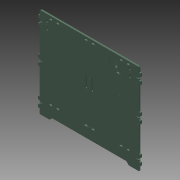
# Autodesk Inventor part: tyl_gt2
Saved by Autodesk Inventor 2013 (Build 170138000, 138)
## iProperties
Created: 2014-01-09
Part Number: tyl_gt2
Material: Generic
Document SubType Name: Modeling
Designer: dzban
Density: 1 g/cm^3
Author: dzban
Autodesk Inventor part; units mm, degrees
ref_plane "YZ Plane" through (0, 0, 0) normal (1, 0, 0) x (0, 1, 0)
ref_plane "XZ Plane" through (0, 0, 0) normal (0, 1, 0) x (-1, 0, 0)
ref_plane "XY Plane" through (0, 0, 0) normal (0, 0, 1) x (1, 0, 0)
sketch "Sketch1" plane through (0, 0, 0) normal (0, 1, 0) x (-1, 0, 0)
  line L0 (126.9556, -58.4026) -> (126.9556, -52.0026)
  line L1 (126.9556, -52.0026) -> (138.8556, -52.0026)
  line L2 (138.8556, -52.0026) -> (138.8556, -58.4026)
  line L3 (138.8556, -58.4026) -> (126.9556, -58.4026)
  arc A0 (161.4486, -20.0075) -> (158.9486, -20.0075) centre (160.1986, -20.0075) ccw
  line L4 (161.4486, -20.0075) -> (161.4486, -40.0075)
  arc A1 (158.9486, -40.0075) -> (161.4486, -40.0075) centre (160.1986, -40.0075) ccw
  line L5 (158.9486, -40.0075) -> (158.9486, -20.0075)
  arc A2 (168.4486, -40.0075) -> (170.9486, -40.0075) centre (169.6986, -40.0075) ccw
  line L6 (168.4486, -40.0075) -> (168.4486, -20.0075)
  arc A3 (170.9486, -20.0075) -> (168.4486, -20.0075) centre (169.6986, -20.0075) ccw
  line L7 (170.9486, -20.0075) -> (170.9486, -40.0075)
  line L8 (261.2986, -171.5221) -> (254.8986, -171.5221)
  line L9 (254.8986, -171.5221) -> (254.8986, -125.0075)
  line L10 (254.8986, -125.0075) -> (261.2986, -125.0075)
  line L11 (261.2986, -125.0075) -> (261.2986, -171.5221)
  line L12 (230.8986, -171.5221) -> (230.8986, -125.0075)
  line L13 (230.8986, -125.0075) -> (237.2986, -125.0075)
  line L14 (237.2986, -125.0075) -> (237.2986, -171.5221)
  line L15 (237.2986, -171.5221) -> (230.8986, -171.5221)
  line L16 (378.2986, -8.4075) -> (366.2986, -8.4075)
  line L17 (366.2986, -8.4075) -> (366.2986, -2.0075)
  line L18 (366.2986, -2.0075) -> (378.2986, -2.0075)
  line L19 (378.2986, -2.0075) -> (378.2986, -8.4075)
  line L20 (405.8986, -8.4075) -> (393.8986, -8.4075)
  line L21 (393.8986, -8.4075) -> (393.8986, -2.0075)
  line L22 (393.8986, -2.0075) -> (405.8986, -2.0075)
  line L23 (405.8986, -2.0075) -> (405.8986, -8.4075)
  line L24 (238.2986, -8.4075) -> (226.2986, -8.4075)
  line L25 (226.2986, -8.4075) -> (226.2986, -2.0075)
  line L26 (226.2986, -2.0075) -> (238.2986, -2.0075)
  line L27 (238.2986, -2.0075) -> (238.2986, -8.4075)
  line L28 (265.8986, -8.4075) -> (253.8986, -8.4075)
  line L29 (253.8986, -8.4075) -> (253.8986, -2.0075)
  line L30 (253.8986, -2.0075) -> (265.8986, -2.0075)
  line L31 (265.8986, -2.0075) -> (265.8986, -8.4075)
  line L32 (98.2986, -8.4075) -> (86.2986, -8.4075)
  line L33 (86.2986, -8.4075) -> (86.2986, -2.0075)
  line L34 (86.2986, -2.0075) -> (98.2986, -2.0075)
  line L35 (98.2986, -2.0075) -> (98.2986, -8.4075)
  line L36 (125.8986, -8.4075) -> (113.8986, -8.4075)
  line L37 (113.8986, -8.4075) -> (113.8986, -2.0075)
  line L38 (113.8986, -2.0075) -> (125.8986, -2.0075)
  line L39 (125.8986, -2.0075) -> (125.8986, -8.4075)
  line L40 (378.2986, -303.4075) -> (366.2986, -303.4075)
  line L41 (366.2986, -303.4075) -> (366.2986, -297.0075)
  line L42 (366.2986, -297.0075) -> (378.2986, -297.0075)
  line L43 (378.2986, -297.0075) -> (378.2986, -303.4075)
  line L44 (405.8986, -303.4075) -> (393.8986, -303.4075)
  line L45 (393.8986, -303.4075) -> (393.8986, -297.0075)
  line L46 (393.8986, -297.0075) -> (405.8986, -297.0075)
  line L47 (405.8986, -297.0075) -> (405.8986, -303.4075)
  line L48 (238.2986, -303.4075) -> (226.2986, -303.4075)
  line L49 (226.2986, -303.4075) -> (226.2986, -297.0075)
  line L50 (226.2986, -297.0075) -> (238.2986, -297.0075)
  line L51 (238.2986, -297.0075) -> (238.2986, -303.4075)
  line L52 (265.8986, -303.4075) -> (253.8986, -303.4075)
  line L53 (253.8986, -303.4075) -> (253.8986, -297.0075)
  line L54 (253.8986, -297.0075) -> (265.8986, -297.0075)
  line L55 (265.8986, -297.0075) -> (265.8986, -303.4075)
  line L56 (98.2986, -303.4075) -> (86.2986, -303.4075)
  line L57 (86.2986, -303.4075) -> (86.2986, -297.0075)
  line L58 (86.2986, -297.0075) -> (98.2986, -297.0075)
  line L59 (98.2986, -297.0075) -> (98.2986, -303.4075)
  line L60 (125.8986, -303.4075) -> (113.8986, -303.4075)
  line L61 (113.8986, -303.4075) -> (113.8986, -297.0075)
  line L62 (113.8986, -297.0075) -> (125.8986, -297.0075)
  line L63 (125.8986, -297.0075) -> (125.8986, -303.4075)
  line L64 (443.6986, -314.9075) -> (436.6986, -314.9075)
  line L65 (436.6986, -314.9075) -> (436.6986, -316.1575)
  line L66 (436.6986, -316.1575) -> (434.8986, -316.1575)
  line L67 (434.8986, -316.1575) -> (434.8986, -314.9075)
  line L68 (434.8986, -314.9075) -> (433.0986, -314.9075)
  line L69 (433.0986, -314.9075) -> (433.0986, -311.9075)
  line L70 (433.0986, -311.9075) -> (434.8986, -311.9075)
  line L71 (434.8986, -311.9075) -> (434.8986, -310.6575)
  line L72 (434.8986, -310.6575) -> (436.6986, -310.6575)
  line L73 (436.6986, -310.6575) -> (436.6986, -311.9075)
  line L74 (436.6986, -311.9075) -> (443.6986, -311.9075)
  line L75 (443.6986, -311.9075) -> (443.6986, -305.8075)
  line L76 (443.6986, -305.8075) -> (449.6986, -305.5075)
  line L77 (449.6986, -305.5075) -> (449.6986, -293.7075)
  line L78 (449.6986, -293.7075) -> (443.6986, -293.4075)
  line L79 (443.6986, -293.4075) -> (443.6986, -189.0075)
  line L80 (443.6986, -189.0075) -> (449.6986, -188.7075)
  line L81 (449.6986, -188.7075) -> (449.6986, -176.9075)
  line L82 (449.6986, -176.9075) -> (443.6986, -176.6075)
  line L83 (443.6986, -176.6075) -> (443.6986, -170.5075)
  line L84 (443.6986, -170.5075) -> (436.6986, -170.5075)
  line L85 (436.6986, -170.5075) -> (436.6986, -171.7575)
  line L86 (436.6986, -171.7575) -> (434.8986, -171.7575)
  line L87 (434.8986, -171.7575) -> (434.8986, -170.5075)
  line L88 (434.8986, -170.5075) -> (433.0986, -170.5075)
  line L89 (433.0986, -170.5075) -> (433.0986, -167.5075)
  line L90 (433.0986, -167.5075) -> (434.8986, -167.5075)
  line L91 (434.8986, -167.5075) -> (434.8986, -166.2575)
  line L92 (434.8986, -166.2575) -> (436.6986, -166.2575)
  line L93 (436.6986, -166.2575) -> (436.6986, -167.5075)
  line L94 (436.6986, -167.5075) -> (443.6986, -167.5075)
  line L95 (443.6986, -167.5075) -> (443.6986, -161.4075)
  line L96 (443.6986, -161.4075) -> (449.6986, -161.1075)
  line L97 (449.6986, -161.1075) -> (449.6986, -149.3075)
  line L98 (449.6986, -149.3075) -> (443.6986, -149.0075)
  line L99 (443.6986, -149.0075) -> (443.6986, -54.0075)
  line L100 (443.6986, -54.0075) -> (449.6986, -53.7075)
  line L101 (449.6986, -53.7075) -> (449.6986, -41.9075)
  line L102 (449.6986, -41.9075) -> (443.6986, -41.6075)
  line L103 (443.6986, -41.6075) -> (443.6986, -35.5075)
  line L104 (443.6986, -35.5075) -> (436.6986, -35.5075)
  line L105 (436.6986, -35.5075) -> (436.6986, -36.7575)
  line L106 (436.6986, -36.7575) -> (434.8986, -36.7575)
  line L107 (434.8986, -36.7575) -> (434.8986, -35.5075)
  line L108 (434.8986, -35.5075) -> (433.0986, -35.5075)
  line L109 (433.0986, -35.5075) -> (433.0986, -32.5075)
  line L110 (433.0986, -32.5075) -> (434.8986, -32.5075)
  line L111 (434.8986, -32.5075) -> (434.8986, -31.2575)
  line L112 (434.8986, -31.2575) -> (436.6986, -31.2575)
  line L113 (436.6986, -31.2575) -> (436.6986, -32.5075)
  line L114 (436.6986, -32.5075) -> (443.6986, -32.5075)
  line L115 (443.6986, -32.5075) -> (443.6986, -26.4075)
  line L116 (443.6986, -26.4075) -> (449.6986, -26.1075)
  line L117 (449.6986, -26.1075) -> (449.6986, -14.3075)
  line L118 (449.6986, -14.3075) -> (443.6986, -14.0075)
  line L119 (443.6986, -14.0075) -> (443.6986, 0.9925)
  arc A4 (443.6986, 0.9925) -> (438.6986, 5.9925) centre (438.6986, 0.9925) ccw
  line L120 (438.6986, 5.9925) -> (53.4986, 5.9925)
  arc A5 (53.4986, 5.9925) -> (48.4986, 0.9925) centre (53.4986, 0.9925) ccw
  line L121 (48.4986, 0.9925) -> (48.4986, -14.0075)
  line L122 (48.4986, -14.0075) -> (42.4986, -14.3075)
  line L123 (42.4986, -14.3075) -> (42.4986, -26.1075)
  line L124 (42.4986, -26.1075) -> (48.4986, -26.4075)
  line L125 (48.4986, -26.4075) -> (48.4986, -32.5075)
  line L126 (48.4986, -32.5075) -> (55.4986, -32.5075)
  line L127 (55.4986, -32.5075) -> (55.4986, -31.2575)
  line L128 (55.4986, -31.2575) -> (57.2986, -31.2575)
  line L129 (57.2986, -31.2575) -> (57.2986, -32.5075)
  line L130 (57.2986, -32.5075) -> (59.0986, -32.5075)
  line L131 (59.0986, -32.5075) -> (59.0986, -35.5075)
  line L132 (59.0986, -35.5075) -> (57.2986, -35.5075)
  line L133 (57.2986, -35.5075) -> (57.2986, -36.7575)
  line L134 (57.2986, -36.7575) -> (55.4986, -36.7575)
  line L135 (55.4986, -36.7575) -> (55.4986, -35.5075)
  line L136 (55.4986, -35.5075) -> (48.4986, -35.5075)
  line L137 (48.4986, -35.5075) -> (48.4986, -41.6075)
  line L138 (48.4986, -41.6075) -> (42.4986, -41.9075)
  line L139 (42.4986, -41.9075) -> (42.4986, -53.7075)
  line L140 (42.4986, -53.7075) -> (48.4986, -54.0075)
  line L141 (48.4986, -54.0075) -> (48.4986, -149.0075)
  line L142 (48.4986, -149.0075) -> (42.4986, -149.3075)
  line L143 (42.4986, -149.3075) -> (42.4986, -161.1075)
  line L144 (42.4986, -161.1075) -> (48.4986, -161.4075)
  line L145 (48.4986, -161.4075) -> (48.4986, -167.5075)
  line L146 (48.4986, -167.5075) -> (55.4986, -167.5075)
  line L147 (55.4986, -167.5075) -> (55.4986, -166.2575)
  line L148 (55.4986, -166.2575) -> (57.2986, -166.2575)
  line L149 (57.2986, -166.2575) -> (57.2986, -167.5075)
  line L150 (57.2986, -167.5075) -> (59.0986, -167.5075)
  line L151 (59.0986, -167.5075) -> (59.0986, -170.5075)
  line L152 (59.0986, -170.5075) -> (57.2986, -170.5075)
  line L153 (57.2986, -170.5075) -> (57.2986, -171.7575)
  line L154 (57.2986, -171.7575) -> (55.4986, -171.7575)
  line L155 (55.4986, -171.7575) -> (55.4986, -170.5075)
  line L156 (55.4986, -170.5075) -> (48.4986, -170.5075)
  line L157 (48.4986, -170.5075) -> (48.4986, -176.6075)
  line L158 (48.4986, -176.6075) -> (42.4986, -176.9075)
  line L159 (42.4986, -176.9075) -> (42.4986, -188.7075)
  line L160 (42.4986, -188.7075) -> (48.4986, -189.0075)
  line L161 (48.4986, -189.0075) -> (48.4986, -293.4075)
  line L162 (48.4986, -293.4075) -> (42.4986, -293.7075)
  line L163 (42.4986, -293.7075) -> (42.4986, -305.5075)
  line L164 (42.4986, -305.5075) -> (48.4986, -305.8075)
  line L165 (48.4986, -305.8075) -> (48.4986, -311.9075)
  line L166 (48.4986, -311.9075) -> (55.4986, -311.9075)
  line L167 (55.4986, -311.9075) -> (55.4986, -310.6575)
  line L168 (55.4986, -310.6575) -> (57.2986, -310.6575)
  line L169 (57.2986, -310.6575) -> (57.2986, -311.9075)
  line L170 (57.2986, -311.9075) -> (59.0986, -311.9075)
  line L171 (59.0986, -311.9075) -> (59.0986, -314.9075)
  line L172 (59.0986, -314.9075) -> (57.2986, -314.9075)
  line L173 (57.2986, -314.9075) -> (57.2986, -316.1575)
  line L174 (57.2986, -316.1575) -> (55.4986, -316.1575)
  line L175 (55.4986, -316.1575) -> (55.4986, -314.9075)
  line L176 (55.4986, -314.9075) -> (48.4986, -314.9075)
  line L177 (48.4986, -314.9075) -> (48.4986, -321.0075)
  line L178 (48.4986, -321.0075) -> (42.4986, -321.3075)
  line L179 (42.4986, -321.3075) -> (42.4986, -333.1075)
  line L180 (42.4986, -333.1075) -> (48.4986, -333.4075)
  line L181 (48.4986, -333.4075) -> (48.4986, -353.4075)
  line L182 (48.4986, -353.4075) -> (88.4986, -353.4075)
  line L183 (88.4986, -353.4075) -> (98.4986, -343.4075)
  line L184 (98.4986, -343.4075) -> (393.6986, -343.4075)
  line L185 (393.6986, -343.4075) -> (403.6986, -353.4075)
  line L186 (403.6986, -353.4075) -> (443.6986, -353.4075)
  line L187 (443.6986, -353.4075) -> (443.6986, -333.4075)
  line L188 (443.6986, -333.4075) -> (449.6986, -333.1075)
  line L189 (449.6986, -333.1075) -> (449.6986, -321.3075)
  line L190 (449.6986, -321.3075) -> (443.6986, -321.0075)
  line L191 (443.6986, -321.0075) -> (443.6986, -314.9075)
  circle A6 centre (425.6986, -61.0075) radius 1.5
  circle A7 centre (66.4986, -61.0075) radius 1.5
  circle A8 centre (57.4986, -52.0075) radius 1.5
  circle A9 centre (434.6986, -52.0075) radius 1.5
  circle A10 centre (106.0986, -300.2075) radius 1.5
  circle A11 centre (246.0986, -300.2075) radius 1.5
  circle A12 centre (386.0986, -300.2075) radius 1.5
  circle A13 centre (106.0986, -5.2075) radius 1.5
  circle A14 centre (246.0986, -5.2075) radius 1.5
  circle A15 centre (386.0986, -5.2075) radius 1.5
  circle A16 centre (246.0986, -132.7575) radius 1.5
  circle A17 centre (246.0986, -154.2575) radius 1.5
  circle A18 centre (140.1628, -36.0853) radius 6
  circle A19 centre (122.9556, -55.2026) radius 1.5
  circle A20 centre (118.4986, -127.4183) radius 1.5
  circle A21 centre (136.1628, -24.0853) radius 1.5
  circle A22 centre (136.1628, -48.0853) radius 1.5
  circle A23 centre (55.4986, -192.4702) radius 1.5
  circle A24 centre (63.4986, -192.4702) radius 1.5
  circle A25 centre (144.1628, -48.0853) radius 1.5
  circle A26 centre (144.1628, -24.0853) radius 1.5
  circle A27 centre (124.9087, -130.187) radius 1.5
  point P0 (0, 0)
  dimension "d0" = 5.9925
  dimension "d1" = 48.4986
  dimension "d2" = 359.4
  dimension "d3" = 395.2
  dimension "d4" = 5
  dimension "d7" = 38.5
  dimension "d8" = 12.4
  dimension "d9" = 6.1
  dimension "d10" = 11.8
  dimension "d11" = 0.3
  dimension "d12" = 6
  dimension "d13" = 3
  dimension "d14" = 7
  dimension "d15" = 1.8
  dimension "d16" = 1.8
  dimension "d17" = 1.25
  dimension "d18" = 1.25
  dimension "d19" = 6.1
  dimension "d20" = 12.4
  dimension "d21" = 135
  dimension "d22" = 6.1
  dimension "d23" = 12.4
  dimension "d24" = 3
  dimension "d25" = 6.1
  dimension "d26" = 12.4
  dimension "d31" = 144.4
  dimension "d32" = 6.1
  dimension "d33" = 12.4
  dimension "d34" = 3
  dimension "d35" = 6.1
  dimension "d36" = 12.4
  dimension "d39" = 11.2
  dimension "d41" = 140
  dimension "d42" = 140
  dimension "d43" = 6.4
  dimension "d44" = 3.2
  dimension "d45" = 3
  dimension "d46" = 12
  dimension "d47" = 7.8
  dimension "d48" = 7.8
  dimension "d49" = 12
  dimension "d50" = 7.8
  dimension "d51" = 7.8
  dimension "d52" = 12
  dimension "d53" = 12
  dimension "d54" = 7.8
  dimension "d55" = 12
  dimension "d56" = 7.8
  dimension "d57" = 12
  dimension "d58" = 53.2
  dimension "d59" = 3.2
  dimension "d61" = 6.4
  dimension "d62" = 6.4
  dimension "d63" = 11.9
  dimension "d64" = 4
  dimension "d65" = 61.1951
  dimension "d66" = 74.457
  dimension "d67" = 3.2
  dimension "d68" = 8
  dimension "d69" = 24
  dimension "d70" = 30.0778
  dimension "d71" = 87.6641
  dimension "d72" = 4
  dimension "d73" = 12
  constraints: 384 end point, 125 parallel, 72 collinear, 28 centre point, 28 tangent, 24 equal radius, 12 point on circle, 11 horizontal alignment, 8 vertical alignment, 6 vertical, 4 horizontal, 1 perpendicular
  measures "d0" distance from line of point (0, 0) L120
  measures "d1" distance from line of point (0, 0) L121
  measures "d2" distance between parallel lines of L120 L182
  measures "d3" distance between parallel lines of L119 L121
  measures "d4" radius of A5
  measures "d7" distance between parallel lines of L120 L126
  measures "d8" distance of L121.end L124.end
  measures "d9" distance of L124.end L125.end
  measures "d10" distance of L122.end L123.end
  measures "d11" vertical distance of L121.end L122.end
  measures "d12" distance between parallel lines of L121 L123
  measures "d13" distance between parallel lines of L126 L136
  measures "d14" distance between parallel lines of L135 L137
  measures "d15" distance from line of L132.end L135
  measures "d16" distance between parallel lines of L131 L133
  measures "d17" distance between parallel lines of L128 L130
  measures "d18" distance between parallel lines of L132 L134
  measures "d19" distance of L136.end L137.end
  measures "d20" distance of L137.end L140.end
  measures "d21" distance between parallel lines of L146 L126
  measures "d22" distance of L144.end L145.end
  measures "d23" distance of L141.end L144.end
  measures "d24" distance between parallel lines of L146 L156
  measures "d25" distance of L156.end L157.end
  measures "d26" distance of L157.end L160.end
  measures "d31" distance between parallel lines of L166 L146
  measures "d32" distance of L164.end L165.end
  measures "d33" distance of L161.end L164.end
  measures "d34" distance between parallel lines of L166 L176
  measures "d35" distance of L176.end L177.end
  measures "d36" distance of L177.end L180.end
  measures "d39" distance from line of L120 A13.centre
  measures "d41" distance of A14.centre A13.centre
  measures "d42" distance of A15.centre A14.centre
  measures "d43" distance between parallel lines of L34 L32
  measures "d44" distance from line of L34 A13.centre
  measures "d45" diameter of A13
  measures "d46" distance between parallel lines of L35 L33
  measures "d47" distance from line of A13.centre L35
  measures "d48" distance from line of L37 A13.centre
  measures "d49" distance between parallel lines of L39 L37
  measures "d50" distance from line of A14.centre L27
  measures "d51" distance from line of L29 A14.centre
  measures "d52" distance between parallel lines of L31 L29
  measures "d53" distance between parallel lines of L25 L27
  measures "d54" distance from line of L21 A15.centre
  measures "d55" distance between parallel lines of L23 L21
  measures "d56" distance from line of L19 A15.centre
  measures "d57" distance between parallel lines of L17 L19
  measures "d58" distance from line of A10.centre L182
  measures "d59" distance from line of A10.centre L56
  measures "d61" distance between parallel lines of L58 L56
  measures "d62" distance between parallel lines of L1 L3
  measures "d63" distance between parallel lines of L2 L0
  measures "d64" distance from line of L0 A19.centre
  measures "d65" distance from line of L120 A19.centre
  measures "d66" distance from line of L141 A19.centre
  measures "d67" distance from line of A19.centre L3
  measures "d68" distance of A25.centre A22.centre
  measures "d69" distance of A26.centre A25.centre
  measures "d70" distance from line of L120 A21.centre
  measures "d71" distance from line of L121 A21.centre
  measures "d72" horizontal distance of A26.centre A18.centre
  measures "d73" vertical distance of A18.centre A26.centre
extrude "Extrusion1" add sketch "Sketch1" along normal blind 6
sketch "Sketch2" plane through (0, 0, 0) normal (0, -1, 0) x (1, 0, 0)
  line L0 (-393.8986, -8.4075) -> (-405.8986, -8.4075) projected
  line L1 (-48.4986, 0.9925) -> (-48.4986, -14.0075) projected
  line L2 (-443.6986, -14.0075) -> (-443.6986, 0.9925) projected
  line L3 (-417.1986, -11.5075) -> (-411.0986, -11.5075)
  line L4 (-411.0986, -11.5075) -> (-411.0986, -23.5075)
  line L5 (-411.0986, -23.5075) -> (-417.1986, -23.5075)
  line L6 (-417.1986, -23.5075) -> (-417.1986, -11.5075)
  line L7 (-88.5986, -11.5075) -> (-82.4986, -11.5075)
  line L8 (-82.4986, -11.5075) -> (-82.4986, -23.5075)
  line L9 (-82.4986, -23.5075) -> (-88.5986, -23.5075)
  line L10 (-88.5986, -23.5075) -> (-88.5986, -11.5075)
  line L11 (-88.5986, -38.5075) -> (-82.4986, -38.5075)
  line L12 (-82.4986, -38.5075) -> (-82.4986, -50.5075)
  line L13 (-82.4986, -50.5075) -> (-88.5986, -50.5075)
  line L14 (-88.5986, -50.5075) -> (-88.5986, -38.5075)
  line L15 (-417.1986, -38.5075) -> (-411.0986, -38.5075)
  line L16 (-411.0986, -38.5075) -> (-411.0986, -50.5075)
  line L17 (-411.0986, -50.5075) -> (-417.1986, -50.5075)
  line L18 (-417.1986, -50.5075) -> (-417.1986, -38.5075)
  circle A0 centre (-414.1486, -31.0075) radius 1.5
  circle A1 centre (-85.5486, -31.0075) radius 1.5
  point P0 (0, 0)
  dimension "d107" = 3
  dimension "d109" = 3
  dimension "d110" = 6.1
  dimension "d111" = 6.1
  dimension "d112" = 12
  dimension "d113" = 12
  dimension "d114" = 15
  dimension "d115" = 7.5
  dimension "d116" = 3.05
  dimension "d117" = 3.05
  dimension "d118" = 26.5
  dimension "d119" = 3.1
  dimension "d120" = 34
  constraints: 32 end point, 8 collinear, 8 parallel, 4 horizontal, 4 perpendicular, 2 centre point, 1 horizontal alignment
  measures "d107" diameter of A0
  measures "d109" diameter of A1
  measures "d110" distance between parallel lines of L16 L18
  measures "d111" distance between parallel lines of L12 L14
  measures "d112" distance between parallel lines of L15 L17
  measures "d113" distance between parallel lines of L3 L5
  measures "d114" distance between parallel lines of L5 L15
  measures "d115" distance from line of A0.centre L15
  measures "d116" distance from line of A0.centre L16
  measures "d117" distance from line of L8 A1.centre
  measures "d118" distance between parallel lines of L2 L6
  measures "d119" distance between parallel lines of L0 L3
  measures "d120" distance between parallel lines of L1 L8
extrude "Extrusion2" cut sketch "Sketch2" against normal blind 10
body "Solid1"
